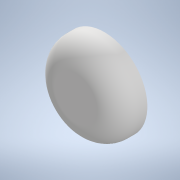
# Autodesk Inventor part: Top_and_Bottom
Saved by Autodesk Inventor 2020.2 (Build 242310000, 310)
## iProperties
Created: 2020-03-04
Part Number: Top_and_Bottom
Material: Generic
Document SubType Name: Modeling
Designer: linus
Density: 1 g/cm^3
Appearance: Default
Author: linus
Autodesk Inventor part; units mm, degrees
ref_plane "YZ Plane" through (0, 0, 0) normal (1, 0, 0) x (0, 1, 0)
ref_plane "XZ Plane" through (0, 0, 0) normal (0, 1, 0) x (-1, 0, 0)
ref_plane "XY Plane" through (0, 0, 0) normal (0, 0, 1) x (1, 0, 0)
sketch "Sketch1" plane through (0, 0, 0) normal (0, 1, 0) x (-1, 0, 0)
  line L0 (0, 0) -> (-30, 0)
  line L1 (-30, 0) -> (-30, 20)
  line L2 (-30, 20) -> (0, 20)
  line L3 (0, 20) -> (0, 0)
  dimension "d0" = 30
  dimension "d1" = 20
  constraints: 8 end point, 2 parallel, 1 horizontal, 1 perpendicular
  measures "d0" distance of L1.end L2.end
  measures "d1" distance of L0.end L1.end
revolve "Revolution1" add sketch "Sketch1" angle 360 about axis through (30, 0, 0) along (0, 0, 1)
fillet "Fillet1" radius 15 1 edges at (60, 0, 20)
body "Solid1"
